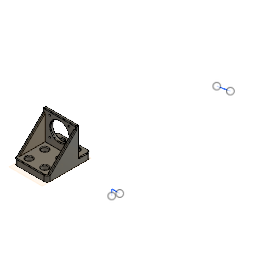
motorMountNema17_v1 (Autodesk Fusion 360 design; units mm, degrees)
Autodesk Fusion 360 part; units mm, degrees
mesh "Mesh1" [no effect]
sketch "Sketch1" plane through (0, 0, 0) normal (0, 1, 0) x (1, 0, 0)
  line L0 (27, 39.5) -> (-27, 39.5)
  line L1 (-27, 39.5) -> (-27, -39.5)
  line L2 (-27, -39.5) -> (27, -39.5)
  line L3 (27, -39.5) -> (27, 39.5)
  line L4 (27, 39.5) -> (-27, -39.5) construction
  line L5 (-27, 39.5) -> (27, -39.5) construction
  dimension "d1" = 54
  dimension "d2" = 79
extrude "Extrude1" add sketch "Sketch1" along normal blind 10
hole "Hole1" at (12.7, 10, -29.7) direction (0, -1, 0) diameter 9.8 depth 7 tip angle 180
hole "Hole2" at (-12.78, 10, -29.7) direction (0, -1, 0) diameter 9.8 depth 7 tip angle 180
hole "Hole3" at (12.7, 0, -29.7) direction (0, 1, 0) diameter 6.1 depth 3 tip angle 180
hole "Hole4" at (-12.7, 0, -29.7) direction (0, 1, 0) diameter 6.1 depth 3 tip angle 180
fillet "Fillet1" radius 1 1 edges at (14.4719, 10, -34.2684)
fillet "Fillet2" radius 1 1 edges at (-11.0081, 10, -34.2684)
sketch "Sketch2" plane through (0, 10, 0) normal (0, 1, 0) x (-1, 0, 0)
  circle A0 centre (-12.7, -29.7) radius 5.9
  line L0 (-27, 39.5) -> (-27, -39.5)
  line L1 (-27, -39.5) -> (27, -39.5)
  line L2 (27, -39.5) -> (27, 39.5)
  line L3 (27, 39.5) -> (-27, 39.5)
  circle A1 centre (12.78, -29.7) radius 5.9
  line L4 (27, -20.1303) -> (-27, -20.1303)
  line L5 (-27, -20.1303) -> (-27, -15.1303)
  line L6 (-27, -15.1303) -> (27, -15.1303)
  line L7 (27, -15.1303) -> (27, -20.1303)
  dimension "d28" = 5
  measures "d28" distance of origin
extrude "Extrude2" add sketch "Sketch2" along normal blind 46.5 contours L0 L2 L4 L5 L6 L7
move_body "Move1" bodies 1 to x (1, 0, 0) y (0, 1, 0) z (0, 0, 1) at (0, -40, 0)
hole "Hole5" at (12.7, -40, -4.3) direction (0, 1, 0) diameter 6.1 depth 3 tip angle 180
hole "Hole6" at (12.7, -40, 21.1) direction (0, 1, 0) diameter 6.1 depth 3 tip angle 180
sketch "Sketch3" plane through (0, -40, 0) normal (0, -1, 0) x (1, 0, 0)
  circle A0 centre (12.7, 21.1) radius 3.05
  circle A1 centre (12.7, -4.3) radius 3.05
  circle A2 centre (-12.7, -29.7) radius 3.05
  circle A3 centre (12.7, -29.7) radius 3.05
  line L0 (27, -39.5) -> (27, 39.5)
  line L1 (27, 39.5) -> (-27, 39.5)
  line L2 (-27, 39.5) -> (-27, -39.5)
  line L3 (-27, -39.5) -> (27, -39.5)
hole "Hole7" at (-12.7, -40, -4.3) direction (0, 1, 0) diameter 6.1 depth 3 tip angle 180
hole "Hole8" at (-12.7, -40, 21.1) direction (0, 1, 0) diameter 6.1 depth 3 tip angle 180
hole "Hole9" at (-12.7, -30, -4.3) direction (0, -1, 0) diameter 9.8 depth 7 tip angle 180
hole "Hole10" at (-12.7, -30, 21.1) direction (0, -1, 0) diameter 9.8 depth 7 tip angle 180
hole "Hole11" at (12.7, -30, -4.3) direction (0, -1, 0) diameter 9.8 depth 7 tip angle 180
hole "Hole12" at (12.7, -30, 21.1) direction (0, -1, 0) diameter 9.8 depth 7 tip angle 180
sketch "Sketch4" plane through (0, -30, 0) normal (0, 1, 0) x (-1, 0, 0)
  circle A0 centre (-12.7, 21.1) radius 4.9
  circle A1 centre (-12.7, -4.3) radius 4.9
  circle A2 centre (12.7, 21.1) radius 4.9
  circle A3 centre (12.7, -4.3) radius 4.9
  line L0 (-27, -15.1303) -> (27, -15.1303)
  line L1 (27, -15.1303) -> (27, 39.5)
  line L2 (27, 39.5) -> (-27, 39.5)
  line L3 (-27, 39.5) -> (-27, -15.1303)
  line L4 (-12.7, 21.1) -> (-12.7, 31.8)
  line L5 (-27, 31.8637) -> (27, 31.8637)
  line L6 (27, 31.8637) -> (27, 39.5)
  line L7 (27, 39.5) -> (-27, 39.5)
  line L8 (-27, 39.5) -> (-27, 31.8637)
  dimension "d71" = 10.7
extrude "Extrude3" cut sketch "Sketch4" against normal blind 12 contours L1 L2 L3 L5 L6 L7 L8
fillet "Fillet3" radius 5 1 edges at (-27, -35, 31.8637)
fillet "Fillet4" radius 5 1 edges at (27, -35, 31.8637)
fillet "Fillet5" radius 5 1 edges at (-27, -35, -39.5)
fillet "Fillet6" radius 5 1 edges at (27, -35, -39.5)
sketch "Sketch5" plane through (0, 0, 0) normal (0, 0, 1) x (1, 0, 0)
sketch "Sketch6" plane through (0, 0, 0) normal (0, 1, 0) x (1, 0, 0)
  line L0 (68, 202) -> (86, 206)
sketch "Sketch7" plane through (0, 0, 0) normal (0, 0, 1) x (1, 0, 0)
  line L0 (100, -27) -> (113, -27)
  line L1 (100, -27) -> (100, -37)
sketch "Sketch8" plane through (0, 0, 0) normal (0, 0, 1) x (1, 0, 0)
hole "Hole13" at (15.5, -20, -20.1303) direction (0, 0, 1) diameter 5.8 depth 3.2 tip angle 180
hole "Hole14" at (-15.5, -20, -20.1303) direction (0, 0, 1) diameter 5.8 depth 3.2 tip angle 180
hole "Hole15" at (15.5, 11, -20.1303) direction (0, 0, 1) diameter 5.8 depth 3.2 tip angle 180
hole "Hole16" at (-15.5, 11, -20.1303) direction (0, 0, 1) diameter 5.8 depth 3.2 tip angle 180
hole "Hole17" at (15.5, -20, -20.1303) direction (0, 0, 1) diameter 2.8 depth 5 tip angle 180
hole "Hole18" at (15.5, 11, -20.1303) direction (0, 0, 1) diameter 2.8 depth 5 tip angle 180
hole "Hole19" at (-15.5, 11, -20.1303) direction (0, 0, 1) diameter 2.8 depth 5 tip angle 180
hole "Hole20" at (-15.5, -20, -20.1303) direction (0, 0, 1) diameter 2.8 depth 5 tip angle 180
chamfer "Chamfer1" distance 0.4 angle 45 1 edges at (-12.7963, 12.0487, -20.1303)
chamfer "Chamfer2" distance 0.4 angle 45 1 edges at (18.2037, 12.0487, -20.1303)
chamfer "Chamfer3" distance 0.4 angle 45 1 edges at (18.2037, -18.9513, -20.1303)
chamfer "Chamfer4" distance 0.4 angle 45 1 edges at (-12.7963, -18.9513, -20.1303)
fillet "Fillet7" radius 1 1 edges at (0, 16.5, -20.1303)
fillet "Fillet8" radius 1 1 edges at (0, 16.5, -15.1303)
hole "Hole21" at (0, -4.5, -20.1303) direction (0, 0, 1) diameter 29 depth 5 tip angle 180
fillet "Fillet9" radius 1 1 edges at (13.5187, 0.7434, -20.1303)
fillet "Fillet10" radius 1 1 edges at (13.5187, -9.7434, -15.1303)
sketch "Sketch9" plane through (-27, 0, 0) normal (-1, 0, 0) x (0, 0, 1)
  arc A0 (-15.1303, 15.5) -> (-16.1303, 16.5) centre (-16.1303, 15.5) ccw
  line L0 (-16.1303, 16.5) -> (-19.1303, 16.5)
  arc A1 (-19.1303, 16.5) -> (-20.1303, 15.5) centre (-19.1303, 15.5) ccw
  line L1 (-20.1303, 15.5) -> (-20.1303, -30)
  line L2 (-20.1303, -30) -> (-34.5, -30)
  line L3 (-34.5, -30) -> (-34.5, -40)
  line L4 (-34.5, -40) -> (26.8637, -40)
  line L5 (26.8637, -40) -> (26.8637, -30)
  line L6 (26.8637, -30) -> (-15.1303, -30)
  line L7 (-15.1303, -30) -> (-15.1303, 15.5)
  line L8 (26.8637, -30) -> (-15.1303, 11)
extrude "Extrude4" add sketch "Sketch9" against normal blind 4 contours L6 L7 L8
sketch "Sketch10" plane through (-23, 0, 0) normal (1, 0, 0) x (0, 0, -1)
  line L0 (-26.8637, -30) -> (15.1303, -30)
  line L1 (15.1303, -30) -> (15.1303, 11)
  line L2 (15.1303, 11) -> (-26.8637, -30)
sketch "Sketch11" plane through (27, 0, 0) normal (1, 0, 0) x (0, 0, -1)
  arc A0 (16.1303, 16.5) -> (15.1303, 15.5) centre (16.1303, 15.5) ccw
  line L0 (15.1303, 15.5) -> (15.1303, -30)
  line L1 (15.1303, -30) -> (-26.8637, -30)
  line L2 (-26.8637, -30) -> (-26.8637, -40)
  line L3 (-26.8637, -40) -> (34.5, -40)
  line L4 (34.5, -40) -> (34.5, -30)
  line L5 (34.5, -30) -> (20.1303, -30)
  line L6 (20.1303, -30) -> (20.1303, 15.5)
  arc A1 (20.1303, 15.5) -> (19.1303, 16.5) centre (19.1303, 15.5) ccw
  line L7 (19.1303, 16.5) -> (16.1303, 16.5)
  line L8 (-26.8637, -30) -> (15.1303, 11)
extrude "Extrude5" add sketch "Sketch11" against normal blind 4 contours L0 L1 L8
fillet "Fillet11" radius 1 1 edges at (-27, -9.5, 5.8667)
fillet "Fillet12" radius 1 1 edges at (-23, -9.5, 5.8667)
fillet "Fillet13" radius 1 1 edges at (27, -9.5, 5.8667)
fillet "Fillet14" radius 1 1 edges at (23, -9.5, 5.8667)
fillet "Fillet15" radius 1 5 edges at (27, -30, 26.1479) (25.5355, -30, 30.3992) (0, -30, 31.8637) (-25.5355, -30, 30.3992) (-27, -30, 26.1479)
fillet "Fillet16" radius 1 5 edges at (27, -30, -27.3151) (25.5355, -30, -38.0355) (0, -30, -39.5) (-25.5355, -30, -38.0355) (-27, -30, -27.3151)
fillet "Fillet17" radius 1 5 edges at (-27, -7.75, -20.1303) (-27, 16.2071, -19.8374) (-27, 16.5, -17.6303) (-27, 16.2071, -15.4232) (-27, 12.5512, -15.1303)
fillet "Fillet18" radius 1 5 edges at (27, -7.75, -20.1303) (27, 16.2071, -19.8374) (27, 16.5, -17.6303) (27, 16.2071, -15.4232) (27, 12.5512, -15.1303)
fillet "Fillet19" radius 1 1 edges at (14.4719, -30, -8.8684)
fillet "Fillet20" radius 1 1 edges at (-10.9281, -30, -8.8684)
fillet "Fillet21" radius 1 1 edges at (-10.9281, -30, 16.5316)
fillet "Fillet22" radius 1 1 edges at (14.4719, -30, 16.5316)
